Autodesk Fusion 360 part; units mm, degrees
(part 2 of 2)
ref_plane "Piano di lavoro7" through (40.5, 0, 0) normal (1, 0, 0) x (0, 1, 0) in component "11_Guscio_fisso_posteriore_torretta_removibile"
sketch "Schizzo7 (6)" plane through (40.5, 0, 0) normal (1, 0, 0) x (0, 0, -1) in component "11_Guscio_fisso_posteriore_torretta_removibile"
  circle A0 centre (-48, -30.3) radius 1.35
extrude "Foro_M2_5_cofano_Destra_01" cut sketch "Schizzo7 (6)" along normal blind 2.5 bodies 16 in component "11_Guscio_fisso_posteriore_torretta_removibile"
ref_plane "Piano di lavoro24" through (36, 0, 0) normal (1, 0, 0) x (0, 1, 0) in component "04_Torretta_parte_fissa_azimut"
sketch "Schizzo29" plane through (36, 0, 0) normal (1, 0, 0) x (0, 0, -1) in component "04_Torretta_parte_fissa_azimut"
  circle A0 centre (-48, -30.3) radius 1.1
extrude "Preforo_M2_5_cofano_telaio_Destra_01" cut sketch "Schizzo29" along normal blind 4 bodies 4 in component "04_Torretta_parte_fissa_azimut"
ref_plane "Piano di lavoro8" through (40.5, 0, 0) normal (1, 0, 0) x (0, 1, 0) in component "11_Guscio_fisso_posteriore_torretta_removibile"
sketch "Schizzo8 (6)" plane through (40.5, 0, 0) normal (1, 0, 0) x (0, 0, -1) in component "11_Guscio_fisso_posteriore_torretta_removibile"
  circle A0 centre (-88, -30.3) radius 1.35
extrude "Foro_M2_5_cofano_Destra_02" cut sketch "Schizzo8 (6)" along normal blind 2.5 bodies 16 in component "11_Guscio_fisso_posteriore_torretta_removibile"
ref_plane "Piano di lavoro25" through (36, 0, 0) normal (1, 0, 0) x (0, 1, 0) in component "04_Torretta_parte_fissa_azimut"
sketch "Schizzo30" plane through (36, 0, 0) normal (1, 0, 0) x (0, 0, -1) in component "04_Torretta_parte_fissa_azimut"
  circle A0 centre (-88, -30.3) radius 1.1
extrude "Preforo_M2_5_cofano_telaio_Destra_02" cut sketch "Schizzo30" along normal blind 4 bodies 4 in component "04_Torretta_parte_fissa_azimut"
ref_plane "Piano di lavoro1" through (-69.5, 0, 0) normal (1, 0, 0) x (0, 1, 0) in component "12_Carter_SG90_Sinistro_removibile"
sketch "Schizzo1 (12)" plane through (-69.5, 0, 0) normal (1, 0, 0) x (0, 0, -1) in component "12_Carter_SG90_Sinistro_removibile"
  line L0 (-65.4, -27.8) -> (-87.1, -27.8)
  line L1 (-87.1, -27.8) -> (-87.1, 16.5)
  line L2 (-87.1, 16.5) -> (-65.4, 16.5)
  line L3 (-65.4, 16.5) -> (-65.4, -27.8)
extrude "Estrusione_Parete_esterna_carter_Sinistro" add sketch "Schizzo1 (12)" along normal blind 2.5 separate body makes body 17 in component "12_Carter_SG90_Sinistro_removibile"
ref_plane "Piano di lavoro2" through (0, -27.8, 0) normal (0, 1, 0) x (0, 0, 1) in component "12_Carter_SG90_Sinistro_removibile"
sketch "Schizzo2 (12)" plane through (0, -27.8, 0) normal (0, 1, 0) x (1, 0, 0) in component "12_Carter_SG90_Sinistro_removibile"
  line L0 (-69.5, -65.4) -> (-40.5, -65.4)
  line L1 (-40.5, -65.4) -> (-40.5, -87.1)
  line L2 (-40.5, -87.1) -> (-69.5, -87.1)
  line L3 (-69.5, -87.1) -> (-69.5, -65.4)
extrude "Estrusione_Parete_Posteriore_carter_Sinistro" add sketch "Schizzo2 (12)" along normal blind 2.5 bodies 17 in component "12_Carter_SG90_Sinistro_removibile"
ref_plane "Piano di lavoro3" through (0, 14, 0) normal (0, 1, 0) x (0, 0, 1) in component "12_Carter_SG90_Sinistro_removibile"
sketch "Schizzo3 (10)" plane through (0, 14, 0) normal (0, 1, 0) x (1, 0, 0) in component "12_Carter_SG90_Sinistro_removibile"
  line L0 (-69.5, -65.4) -> (-40.5, -65.4)
  line L1 (-40.5, -65.4) -> (-40.5, -87.1)
  line L2 (-40.5, -87.1) -> (-69.5, -87.1)
  line L3 (-69.5, -87.1) -> (-69.5, -65.4)
extrude "Estrusione_Parete_Anteriore_carter_Sinistro" add sketch "Schizzo3 (10)" along normal blind 2.5 bodies 17 in component "12_Carter_SG90_Sinistro_removibile"
ref_plane "Piano di lavoro4" through (0, 0, 84.6) normal (0, 0, 1) x (1, 0, 0) in component "12_Carter_SG90_Sinistro_removibile"
sketch "Schizzo4 (9)" plane through (0, 0, 84.6) normal (0, 0, 1) x (1, 0, 0) in component "12_Carter_SG90_Sinistro_removibile"
  line L0 (-69.5, -27.8) -> (-40.5, -27.8)
  line L1 (-40.5, -27.8) -> (-40.5, 16.5)
  line L2 (-40.5, 16.5) -> (-69.5, 16.5)
  line L3 (-69.5, 16.5) -> (-69.5, -27.8)
extrude "Estrusione_Tetto_carter_Sinistro" add sketch "Schizzo4 (9)" along normal blind 2.5 bodies 17 in component "12_Carter_SG90_Sinistro_removibile"
ref_plane "Piano di lavoro5" through (-69.5, 0, 0) normal (1, 0, 0) x (0, 1, 0) in component "12_Carter_SG90_Sinistro_removibile"
sketch "Schizzo5 (7)" plane through (-69.5, 0, 0) normal (1, 0, 0) x (0, 0, -1) in component "12_Carter_SG90_Sinistro_removibile"
  circle A0 centre (-75, -23.55) radius 1.35
extrude "Foro_M2_5_carter_Sinistro_01" cut sketch "Schizzo5 (7)" along normal blind 2.5 bodies 17 in component "12_Carter_SG90_Sinistro_removibile"
ref_plane "Piano di lavoro6" through (-69.5, 0, 0) normal (1, 0, 0) x (0, 1, 0) in component "12_Carter_SG90_Sinistro_removibile"
sketch "Schizzo6 (7)" plane through (-69.5, 0, 0) normal (1, 0, 0) x (0, 0, -1) in component "12_Carter_SG90_Sinistro_removibile"
  circle A0 centre (-75, 12.25) radius 1.35
extrude "Foro_M2_5_carter_Sinistro_02" cut sketch "Schizzo6 (7)" along normal blind 2.5 bodies 17 in component "12_Carter_SG90_Sinistro_removibile"
ref_plane "Piano di lavoro1" through (67, 0, 0) normal (1, 0, 0) x (0, 1, 0) in component "13_Carter_SG90_Destro_removibile"
sketch "Schizzo1 (13)" plane through (67, 0, 0) normal (1, 0, 0) x (0, 0, -1) in component "13_Carter_SG90_Destro_removibile"
  line L0 (-65.4, -27.8) -> (-87.1, -27.8)
  line L1 (-87.1, -27.8) -> (-87.1, 16.5)
  line L2 (-87.1, 16.5) -> (-65.4, 16.5)
  line L3 (-65.4, 16.5) -> (-65.4, -27.8)
extrude "Estrusione_Parete_esterna_carter_Destro" add sketch "Schizzo1 (13)" along normal blind 2.5 separate body makes body 18 in component "13_Carter_SG90_Destro_removibile"
ref_plane "Piano di lavoro2" through (0, -27.8, 0) normal (0, 1, 0) x (0, 0, 1) in component "13_Carter_SG90_Destro_removibile"
sketch "Schizzo2 (13)" plane through (0, -27.8, 0) normal (0, 1, 0) x (1, 0, 0) in component "13_Carter_SG90_Destro_removibile"
  line L0 (40.5, -65.4) -> (69.5, -65.4)
  line L1 (69.5, -65.4) -> (69.5, -87.1)
  line L2 (69.5, -87.1) -> (40.5, -87.1)
  line L3 (40.5, -87.1) -> (40.5, -65.4)
extrude "Estrusione_Parete_Posteriore_carter_Destro" add sketch "Schizzo2 (13)" along normal blind 2.5 bodies 18 in component "13_Carter_SG90_Destro_removibile"
ref_plane "Piano di lavoro3" through (0, 14, 0) normal (0, 1, 0) x (0, 0, 1) in component "13_Carter_SG90_Destro_removibile"
sketch "Schizzo3 (11)" plane through (0, 14, 0) normal (0, 1, 0) x (1, 0, 0) in component "13_Carter_SG90_Destro_removibile"
  line L0 (40.5, -65.4) -> (69.5, -65.4)
  line L1 (69.5, -65.4) -> (69.5, -87.1)
  line L2 (69.5, -87.1) -> (40.5, -87.1)
  line L3 (40.5, -87.1) -> (40.5, -65.4)
extrude "Estrusione_Parete_Anteriore_carter_Destro" add sketch "Schizzo3 (11)" along normal blind 2.5 bodies 18 in component "13_Carter_SG90_Destro_removibile"
ref_plane "Piano di lavoro4" through (0, 0, 84.6) normal (0, 0, 1) x (1, 0, 0) in component "13_Carter_SG90_Destro_removibile"
sketch "Schizzo4 (10)" plane through (0, 0, 84.6) normal (0, 0, 1) x (1, 0, 0) in component "13_Carter_SG90_Destro_removibile"
  line L0 (40.5, -27.8) -> (69.5, -27.8)
  line L1 (69.5, -27.8) -> (69.5, 16.5)
  line L2 (69.5, 16.5) -> (40.5, 16.5)
  line L3 (40.5, 16.5) -> (40.5, -27.8)
extrude "Estrusione_Tetto_carter_Destro" add sketch "Schizzo4 (10)" along normal blind 2.5 bodies 18 in component "13_Carter_SG90_Destro_removibile"
ref_plane "Piano di lavoro5" through (67, 0, 0) normal (1, 0, 0) x (0, 1, 0) in component "13_Carter_SG90_Destro_removibile"
sketch "Schizzo5 (8)" plane through (67, 0, 0) normal (1, 0, 0) x (0, 0, -1) in component "13_Carter_SG90_Destro_removibile"
  circle A0 centre (-75, -23.55) radius 1.35
extrude "Foro_M2_5_carter_Destro_01" cut sketch "Schizzo5 (8)" along normal blind 2.5 bodies 18 in component "13_Carter_SG90_Destro_removibile"
ref_plane "Piano di lavoro6" through (67, 0, 0) normal (1, 0, 0) x (0, 1, 0) in component "13_Carter_SG90_Destro_removibile"
sketch "Schizzo6 (8)" plane through (67, 0, 0) normal (1, 0, 0) x (0, 0, -1) in component "13_Carter_SG90_Destro_removibile"
  circle A0 centre (-75, 12.25) radius 1.35
extrude "Foro_M2_5_carter_Destro_02" cut sketch "Schizzo6 (8)" along normal blind 2.5 bodies 18 in component "13_Carter_SG90_Destro_removibile"
ref_plane "Piano di lavoro1" through (0, 0, 77) normal (0, 0, 1) x (1, 0, 0) in component "14_Guscio_mobile_cannone_removibile"
sketch "Schizzo1 (14)" plane through (0, 0, 77) normal (0, 0, 1) x (1, 0, 0) in component "14_Guscio_mobile_cannone_removibile"
  line L0 (-28, -13) -> (-25.5, -13)
  line L1 (-25.5, -13) -> (-25.5, 43)
  line L2 (-25.5, 43) -> (-28, 43)
  line L3 (-28, 43) -> (-28, -13)
extrude "Estrusione_Parete_mobile_Ovest" add sketch "Schizzo1 (14)" along normal blind 26 separate body makes body 19 in component "14_Guscio_mobile_cannone_removibile"
sketch "Schizzo2 (14)" plane through (0, 0, 77) normal (0, 0, 1) x (1, 0, 0) in component "14_Guscio_mobile_cannone_removibile"
  line L0 (-28, -13) -> (28, -13)
  line L1 (28, -13) -> (28, -10.5)
  line L2 (28, -10.5) -> (-28, -10.5)
  line L3 (-28, -10.5) -> (-28, -13)
extrude "Estrusione_Parete_mobile_Posteriore" add sketch "Schizzo2 (14)" along normal blind 26 bodies 19 in component "14_Guscio_mobile_cannone_removibile"
sketch "Schizzo3 (12)" plane through (0, 0, 77) normal (0, 0, 1) x (1, 0, 0) in component "14_Guscio_mobile_cannone_removibile"
  line L0 (25.5, -13) -> (28, -13)
  line L1 (28, -13) -> (28, 43)
  line L2 (28, 43) -> (25.5, 43)
  line L3 (25.5, 43) -> (25.5, -13)
extrude "Estrusione_Parete_mobile_Est" add sketch "Schizzo3 (12)" along normal blind 26 bodies 19 in component "14_Guscio_mobile_cannone_removibile"
sketch "Schizzo4 (11)" plane through (0, 0, 77) normal (0, 0, 1) x (1, 0, 0) in component "14_Guscio_mobile_cannone_removibile"
  line L0 (-28, 40.5) -> (28, 40.5)
  line L1 (28, 40.5) -> (28, 43)
  line L2 (28, 43) -> (-28, 43)
  line L3 (-28, 43) -> (-28, 40.5)
extrude "Estrusione_Parete_mobile_Anteriore" add sketch "Schizzo4 (11)" along normal blind 26 bodies 19 in component "14_Guscio_mobile_cannone_removibile"
ref_plane "Piano di lavoro2" through (0, 0, 100.5) normal (0, 0, 1) x (1, 0, 0) in component "14_Guscio_mobile_cannone_removibile"
sketch "Schizzo5 (9)" plane through (0, 0, 100.5) normal (0, 0, 1) x (1, 0, 0) in component "14_Guscio_mobile_cannone_removibile"
  line L0 (-28, -13) -> (28, -13)
  line L1 (28, -13) -> (28, 43)
  line L2 (28, 43) -> (-28, 43)
  line L3 (-28, 43) -> (-28, -13)
extrude "Estrusione_Tetto_guscio_mobile_cannone" add sketch "Schizzo5 (9)" along normal blind 2.5 bodies 19 in component "14_Guscio_mobile_cannone_removibile"
ref_plane "Piano di lavoro3" through (0, 40.5, 0) normal (0, 1, 0) x (0, 0, 1) in component "14_Guscio_mobile_cannone_removibile"
sketch "Schizzo6 (9)" plane through (0, 40.5, 0) normal (0, 1, 0) x (1, 0, 0) in component "14_Guscio_mobile_cannone_removibile"
  circle A0 centre (0, -90) radius 5.5
extrude "Passaggio_canna_guscio_mobile_diametro_11" cut sketch "Schizzo6 (9)" along normal blind 2.5 bodies 15 makes body 20 at (4.9752, 36.1667, 89.5022) in component "10_Modulo_cannone_reale_PCB_solenoide_canna"
extrude "Estrusione6" cut sketch "Schizzo6 (9)" along normal blind 2.5 bodies 19 in component "14_Guscio_mobile_cannone_removibile"
ref_plane "Piano di lavoro4" through (0, 40.5, 0) normal (0, 1, 0) x (0, 0, 1) in component "14_Guscio_mobile_cannone_removibile"
sketch "Schizzo7 (7)" plane through (0, 40.5, 0) normal (0, 1, 0) x (1, 0, 0) in component "14_Guscio_mobile_cannone_removibile"
  line L0 (-5.5, -77) -> (5.5, -77)
  line L1 (5.5, -77) -> (5.5, -90)
  line L2 (5.5, -90) -> (-5.5, -90)
  line L3 (-5.5, -90) -> (-5.5, -77)
extrude "Cava_U_inferiore_smontaggio_guscio_mobile" cut sketch "Schizzo7 (7)" along normal blind 2.5 bodies 19 in component "14_Guscio_mobile_cannone_removibile"
ref_plane "Piano di lavoro5" through (0, -13, 0) normal (0, 1, 0) x (0, 0, 1) in component "14_Guscio_mobile_cannone_removibile"
sketch "Schizzo8 (7)" plane through (0, -13, 0) normal (0, 1, 0) x (1, 0, 0) in component "14_Guscio_mobile_cannone_removibile"
  line L0 (-3, -77) -> (3, -77)
  line L1 (3, -77) -> (3, -81)
  line L2 (3, -81) -> (-3, -81)
  line L3 (-3, -81) -> (-3, -77)
extrude "Tacca_posteriore_cavo_cannone_aperta_inferiormente" cut sketch "Schizzo8 (7)" along normal blind 2.5 bodies 19 in component "14_Guscio_mobile_cannone_removibile"
ref_plane "Piano di lavoro6" through (0, 0, 79) normal (0, 0, 1) x (1, 0, 0) in component "14_Guscio_mobile_cannone_removibile"
sketch "Schizzo9 (6)" plane through (0, 0, 79) normal (0, 0, 1) x (1, 0, 0) in component "14_Guscio_mobile_cannone_removibile"
  circle A0 centre (-20, -5) radius 5
extrude "Estrusione_Colonna_M3_guscio_mobile_01" add sketch "Schizzo9 (6)" along normal blind 21.7 bodies 19 in component "14_Guscio_mobile_cannone_removibile"
sketch "Schizzo10 (6)" plane through (0, 0, 79) normal (0, 0, 1) x (1, 0, 0) in component "14_Guscio_mobile_cannone_removibile"
  circle A0 centre (-20, -5) radius 1.75
extrude "Foro_M3_guscio_mobile_01" cut sketch "Schizzo10 (6)" along normal blind 24 bodies 19 in component "14_Guscio_mobile_cannone_removibile"
sketch "Schizzo11 (5)" plane through (0, 0, 79) normal (0, 0, 1) x (1, 0, 0) in component "14_Guscio_mobile_cannone_removibile"
  circle A0 centre (20, -5) radius 5
extrude "Estrusione_Colonna_M3_guscio_mobile_02" add sketch "Schizzo11 (5)" along normal blind 21.7 bodies 19 in component "14_Guscio_mobile_cannone_removibile"
sketch "Schizzo12 (4)" plane through (0, 0, 79) normal (0, 0, 1) x (1, 0, 0) in component "14_Guscio_mobile_cannone_removibile"
  circle A0 centre (20, -5) radius 1.75
extrude "Foro_M3_guscio_mobile_02" cut sketch "Schizzo12 (4)" along normal blind 24 bodies 19 in component "14_Guscio_mobile_cannone_removibile"
sketch "Schizzo13 (4)" plane through (0, 0, 79) normal (0, 0, 1) x (1, 0, 0) in component "14_Guscio_mobile_cannone_removibile"
  circle A0 centre (-20, 35) radius 5
extrude "Estrusione_Colonna_M3_guscio_mobile_03" add sketch "Schizzo13 (4)" along normal blind 21.7 bodies 19 in component "14_Guscio_mobile_cannone_removibile"
sketch "Schizzo14 (4)" plane through (0, 0, 79) normal (0, 0, 1) x (1, 0, 0) in component "14_Guscio_mobile_cannone_removibile"
  circle A0 centre (-20, 35) radius 1.75
extrude "Foro_M3_guscio_mobile_03" cut sketch "Schizzo14 (4)" along normal blind 24 bodies 19 in component "14_Guscio_mobile_cannone_removibile"
sketch "Schizzo15 (3)" plane through (0, 0, 79) normal (0, 0, 1) x (1, 0, 0) in component "14_Guscio_mobile_cannone_removibile"
  circle A0 centre (20, 35) radius 5
extrude "Estrusione_Colonna_M3_guscio_mobile_04" add sketch "Schizzo15 (3)" along normal blind 21.7 bodies 19 in component "14_Guscio_mobile_cannone_removibile"
sketch "Schizzo16 (3)" plane through (0, 0, 79) normal (0, 0, 1) x (1, 0, 0) in component "14_Guscio_mobile_cannone_removibile"
  circle A0 centre (20, 35) radius 1.75
extrude "Foro_M3_guscio_mobile_04" cut sketch "Schizzo16 (3)" along normal blind 24 bodies 19 in component "14_Guscio_mobile_cannone_removibile"
sketch "Schizzo1 (15)" plane through (0, 0, 0) normal (0, 1, 0) x (1, 0, 0)
  line L0 (0, -20) -> (0, 20)
ref_plane "Piano di lavoro1" through (0, 0, 75) normal (0, 0, 1) x (1, 0, 0)
sketch "Schizzo2 (15)" plane through (0, 0, 75) normal (0, 0, 1) x (1, 0, 0)
  line L0 (-20, 0) -> (20, 0)
component "01_Tetto_elettronica_removibile" placed x (1, 0, 0) y (0, 1, 0) z (0, 0, 1) at (0, 0, 0)
component "02_Stepper_28BYJ48_riferimento" placed x (1, 0, 0) y (0, 1, 0) z (0, 0, 1) at (0, 0, 0)
component "03_Adattatore_rotante_stepper" placed x (1, 0, 0) y (0, 1, 0) z (0, 0, 1) at (0, 0, 0)
component "04_Torretta_parte_fissa_azimut" placed x (1, 0, 0) y (0, 1, 0) z (0, 0, 1) at (0, 0, 0)
component "05_Servo_TowerPro_SG90_Sinistro_riferimento" placed x (1, 0, 0) y (0, 1, 0) z (0, 0, 1) at (0, 0, 0)
component "06_Servo_TowerPro_SG90_Destro_riferimento" placed x (1, 0, 0) y (0, 1, 0) z (0, 0, 1) at (0, 0, 0)
component "07_Barrette_removibili_M2_5_SG90_Sinistra" placed x (1, 0, 0) y (0, 1, 0) z (0, 0, 1) at (0, 0, 0)
component "08_Barrette_removibili_M2_5_SG90_Destra" placed x (1, 0, 0) y (0, 1, 0) z (0, 0, 1) at (0, 0, 0)
component "09_Torretta_parte_mobile_elevazione" placed x (1, 0, 0) y (0, 1, 0) z (0, 0, 1) at (0, 0, 0)
component "10_Modulo_cannone_reale_PCB_solenoide_canna" placed x (1, 0, 0) y (0, 1, 0) z (0, 0, 1) at (0, 0, 0)
component "11_Guscio_fisso_posteriore_torretta_removibile" placed x (1, 0, 0) y (0, 1, 0) z (0, 0, 1) at (0, 0, 0)
component "12_Carter_SG90_Sinistro_removibile" placed x (1, 0, 0) y (0, 1, 0) z (0, 0, 1) at (0, 0, 0)
component "13_Carter_SG90_Destro_removibile" placed x (1, 0, 0) y (0, 1, 0) z (0, 0, 1) at (0, 0, 0)
component "14_Guscio_mobile_cannone_removibile" placed x (1, 0, 0) y (0, 1, 0) z (0, 0, 1) at (0, 0, 0)
equation "cop_lunghezza = 176.0 mm" comment "Ingombro coperchio"
equation "cop_larghezza = 166.0 mm" comment "Ingombro coperchio"
equation "cop_parete_altezza = 30.0 mm" comment "Quota locale del tetto removibile"
equation "cop_tetto_spessore = 3.0 mm" comment "Coperchio elettronica"
equation "cop_boss_M3_diametro = 10.0 mm" comment "Accesso vite M3 dal tetto alle colonnine"
equation "cop_razza_supporto_raggio_interno = 19.0 mm" comment "Supporto ribassato disco stepper"
equation "cop_razza_supporto_raggio_esterno = 37.0 mm" comment "Supporto ribassato disco stepper"
equation "cop_razza_supporto_larghezza = 5.0 mm" comment "Supporto ribassato disco stepper"
equation "cop_razza_supporto_spessore = 3.0 mm" comment "Supporto ribassato disco stepper"
equation "stepper_corpo_diametro = 28.0 mm" comment "Riferimento stepper"
equation "stepper_corpo_altezza = 20.0 mm" comment "Riferimento stepper"
equation "stepper_albero_diametro = 5.0 mm" comment "Riferimento stepper"
equation "stepper_albero_lunghezza = 9.0 mm" comment "Riferimento stepper"
equation "stepper_interasse_fori = 35.0 mm" comment "Fissaggio stepper"
equation "stepper_foro_fissaggio = 4.2 mm" comment "Fissaggio stepper"
equation "torre_base_diametro = 70.0 mm" comment "Adattatore rotante"
equation "torre_base_spessore = 6.0 mm" comment "Adattatore rotante"
equation "torre_fissa_larghezza = 80.0 mm" comment "Parte fissa torretta"
equation "torre_fissa_lunghezza = 70.0 mm" comment "Parte fissa torretta"
equation "torre_fissa_altezza = 50.0 mm" comment "Parte fissa torretta"
equation "torre_parete_spessore = 4.0 mm" comment "Parte fissa torretta"
equation "torre_perno_quota = 32.0 mm" comment "Asse elevazione"
equation "servo_corpo_lunghezza = 22.7 mm" comment "TowerPro SG90"
equation "servo_corpo_larghezza = 12.2 mm" comment "TowerPro SG90"
equation "servo_corpo_altezza = 27.0 mm" comment "TowerPro SG90"
equation "servo_ingombro_con_uscita = 30.3 mm" comment "TowerPro SG90"
equation "servo_alette_lunghezza_totale = 32.3 mm" comment "TowerPro SG90"
equation "servo_asse_da_estremita = 17.0 mm" comment "TowerPro SG90"
equation "servo_albero_sporgenza = 3.3 mm" comment "TowerPro SG90"
equation "servo_perno_diametro = 6.0 mm" comment "Perni servo coassiali"
equation "servo_gioco_inserimento = 0.5 mm" comment "Slitta servo"
equation "servo_supporto_parete = 2.5 mm" comment "Slitta servo"
equation "servo_supporto_ripiano = 2.5 mm" comment "Slitta servo"
equation "servo_barretta_spessore = 3.0 mm" comment "Chiusura removibile servo"
equation "servo_barretta_sovrapposizione = 3.0 mm" comment "Chiusura removibile servo"
equation "servo_foro_M2_5 = 2.7 mm" comment "Chiusura removibile servo"
equation "servo_preforo_M2_5 = 2.2 mm" comment "Slitta servo"
equation "servo_cavo_larghezza = 4.0 mm" comment "Cavo piatto SG90"
equation "servo_cavo_spessore = 1.0 mm" comment "Cavo piatto SG90"
equation "servo_uscita_cavo_larghezza = 5.0 mm" comment "Slitta SG90"
equation "servo_uscita_cavo_profondita = 2.0 mm" comment "Slitta SG90"
equation "servo_connettore_larghezza = 7.0 mm" comment "Connettore SG90"
equation "servo_connettore_spessore = 3.0 mm" comment "Connettore SG90"
equation "passaggio_comune_larghezza = 8.0 mm" comment "Passaggio connettori SG90"
equation "passaggio_comune_lunghezza = 6.0 mm" comment "Passaggio connettori SG90"
equation "passaggio_arco_raggio = 28.0 mm" comment "Guida cavi azimut"
equation "passaggio_arco_larghezza = 8.0 mm" comment "Guida cavi azimut"
equation "cannone_connettore_larghezza = 5.0 mm" comment "Connettore cannone"
equation "cannone_connettore_spessore = 3.0 mm" comment "Connettore cannone"
equation "cannone_passaggio_mobile_larghezza = 6.0 mm" comment "Passaggio sotto culla"
equation "cannone_passaggio_mobile_lunghezza = 4.0 mm" comment "Passaggio sotto culla"
equation "pcb_cannone_lunghezza = 50.0 mm" comment "PCB mobile cannone"
equation "pcb_cannone_larghezza = 50.0 mm" comment "PCB mobile cannone"
equation "pcb_cannone_spessore = 2.0 mm" comment "PCB mobile cannone"
equation "pcb_cannone_foro = 3.5 mm" comment "Fori PCB cannone"
equation "pcb_cannone_foro_bordo_x = 5.0 mm" comment "Fori PCB cannone"
equation "pcb_cannone_foro_bordo_y = 5.0 mm" comment "Fori PCB cannone"
equation "solenoide_diametro = 20.0 mm" comment "Zona solenoide"
equation "solenoide_lunghezza = 25.0 mm" comment "Zona solenoide"
equation "canna_diametro_esterno = 10.0 mm" comment "Canna tubolare"
equation "canna_diametro_interno = 8.0 mm" comment "Canna tubolare"
equation "canna_parete = 1.0 mm" comment "Canna tubolare"
equation "canna_sporgenza = 46.0 mm" comment "Canna tubolare"
equation "modulo_cannone_altezza = 23.0 mm" comment "Modulo mobile"
equation "cannone_elevazione_min = -10.0 deg" comment "Limite proposto asse elevazione"
equation "cannone_elevazione_max = 35.0 deg" comment "Limite proposto asse elevazione"
equation "passaggio_arco_angolo_iniziale = 0.0 deg" comment "Inizio guida cavi di azimut"
equation "passaggio_arco_corsa = 360.0 deg" comment "Corsa totale guida cavi di azimut"
equation "torretta_azimut_min = -180.0 deg" comment "Limite software e giunto Fusion"
equation "torretta_azimut_max = 180.0 deg" comment "Limite software e giunto Fusion"
equation "d71 = cop_parete_altezza"
equation "d73 = cop_tetto_spessore"
equation "d91 = cop_parete_altezza"
equation "d93 = cop_tetto_spessore"
equation "d95 = cop_tetto_spessore"
equation "d97 = cop_tetto_spessore"
equation "d125 = cop_tetto_spessore"
equation "d129 = stepper_corpo_altezza"
equation "d137 = stepper_albero_lunghezza"
equation "d141 = torre_base_spessore"
equation "d143 = torre_base_spessore"
equation "d145 = torre_base_spessore"
equation "d149 = torre_base_spessore"
equation "d153 = torre_base_spessore"
equation "d157 = torre_base_spessore"
equation "d161 = torre_base_spessore"
equation "d165 = torre_base_spessore"
equation "d263 = servo_corpo_altezza"
equation "d267 = servo_albero_sporgenza"
equation "d271 = servo_corpo_altezza"
equation "d275 = servo_albero_sporgenza"
equation "d279 = servo_barretta_spessore"
equation "d283 = servo_barretta_spessore"
equation "d287 = servo_barretta_spessore"
equation "d291 = servo_barretta_spessore"
equation "d295 = servo_barretta_spessore"
equation "d299 = servo_barretta_spessore"
equation "d303 = servo_barretta_spessore"
equation "d307 = servo_barretta_spessore"
equation "d349 = pcb_cannone_spessore"
equation "d351 = pcb_cannone_spessore"
equation "d353 = pcb_cannone_spessore"
equation "d355 = pcb_cannone_spessore"
equation "d357 = pcb_cannone_spessore"
equation "d365 = solenoide_lunghezza"
equation "d369 = solenoide_lunghezza"
equation "d373 = canna_sporgenza"
equation "d377 = canna_sporgenza"
equation "guscio_torretta_parete = 2.5 mm" comment "Gusci removibili torretta"
equation "guscio_torretta_gioco = 0.5 mm" comment "Gioco attorno a telaio, servo e modulo mobile"
equation "guscio_cannone_foro_canna = 11.0 mm" comment "Passaggio canna nel guscio mobile"
named bodies: "Tetto_removibile_con_supporto_stepper_e_boss_M3", "Corpo_stepper", "Piastra_adattatore_rotante", "Base_parte_fissa", "Corpo_SG90_Sinistro", "Corpo_SG90_Destro", "Barretta_Sinistra_01", "Barretta_Sinistra_02", "Barretta_Destra_01", "Barretta_Destra_02", "Piastra_culla_mobile", "PCB_modulo_cannone_50x50", "Appoggio_solenoide_su_PCB", "Corpo_solenoide_riferimento", "Canna_tubolare_esterna", "Parete_posteriore_guscio_torretta", "Parete_esterna_carter_Sinistro", "Parete_esterna_carter_Destro", "Parete_mobile_Ovest", "Canna_tubolare_esterna (1)"
